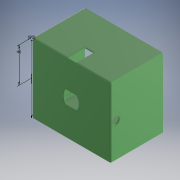
# Autodesk Inventor part: corps
Saved by Autodesk Inventor 2017 (Build 210142000, 142)
## iProperties
Part Number: corps
Material: Plastique ABS
Document SubType Name: Modeling
Designer: starl
Density: 1.06 g/cm^3
Appearance: Lisse - Blanc
Author: starl
Autodesk Inventor part; units mm, degrees
ref_plane "YZ Plane" through (0, 0, 0) normal (1, 0, 0) x (0, 1, 0)
ref_plane "XZ Plane" through (0, 0, 0) normal (0, 1, 0) x (-1, 0, 0)
ref_plane "XY Plane" through (0, 0, 0) normal (0, 0, 1) x (1, 0, 0)
sketch "Esquisse1" plane through (0, 0, 0) normal (1, 0, 0) x (0, 1, 0)
  line L0 (0, 0) -> (60, 0)
  line L1 (60, 0) -> (60, -80)
  line L2 (60, -80) -> (0, -80)
  line L3 (0, -80) -> (0, 0)
  line L4 (0, -45) -> (0, -35)
  line L5 (0, -35) -> (0, -45)
  point P0 (12.5, -45)
  point P1 (0, -40)
  point P2 (0, -40)
  dimension "d0" = 80
  dimension "d1" = 60
  dimension "d4" = 40
  constraints: 12 end point, 3 equal length, 3 midpoint, 1 horizontal, 1 perpendicular, 1 point on line
  measures "d0" distance of L0.end L1.end
  measures "d1" distance of L1.end L2.end
  measures "d4" distance of point (0, -40) L2.end
extrude "Extrusion1" add sketch "Esquisse1" along normal blind 90
sketch "Esquisse2" plane through (0, 0, 0) normal (-1, 0, 0) x (0, 0, 1)
  line L0 (0, 0) -> (-80, 0) projected
  line L1 (-45, 0) -> (-35, 0)
  line L2 (0, 0) -> (-80, 0) projected
  point P0 (-40, 0)
  point P1 (-40, 0)
  point P2 (-40, 1)
  point P3 (-41.0501, 0)
  point P4 (-35, 9.6008)
  point P5 (-45, 11)
  dimension "d9" = 40
  dimension "d14" = 80
  constraints: 3 midpoint, 2 end point, 2 point on line, 2 vertical alignment, 1 coincident, 1 horizontal
  measures "d9" distance of L0.start point (-40, 0)
  measures "d14" distance of L0.start L0.end
shell "Coque1" thickness 1 removed faces 1 at (30, 60, -53.3333)
sketch "Esquisse3" plane through (0, 0, 0) normal (-1, 0, 0) x (0, 0, 1)
  point P0 (0, 0)
sketch "Esquisse4" plane through (0, 0, 0) normal (-1, 0, 0) x (0, 0, 1)
  point P0 (0, 0)
sketch "Esquisse5" plane through (0, 0, -80) normal (0, 0, -1) x (-1, 0, 0)
  line L0 (-50.2889, 1) -> (-40.2889, 1)
  line L1 (-40.2889, 1) -> (-40.2889, 21)
  line L2 (-40.2889, 21) -> (-50.2889, 21)
  line L3 (-50.2889, 21) -> (-50.2889, 1)
  line L4 (0, 0) -> (-90, 0) projected
  line L5 (0, 0) -> (-90, 0) projected
  line L6 (-1, 1) -> (-89, 1) projected
  point P0 (-45, 0)
  point P1 (-40.2889, 0)
  point P2 (-49.4557, 1)
  point P3 (-46.3284, -7.001)
  point P4 (-44.591, 0)
  point P5 (-46.3284, -7.537)
  point P6 (-50.2889, 11)
  point P7 (-50.2889, 11)
  point P8 (-49.5179, 0)
  point P9 (-49.2163, 0)
  dimension "d15" = 10
  dimension "d16" = 20
  dimension "d17" = 1
  dimension "d18" = 88
  dimension "d19" = 90
  constraints: 8 end point, 6 point on line, 2 midpoint, 2 parallel, 1 coincident, 1 horizontal, 1 perpendicular
  measures "d15" distance of L1.end L2.end
  measures "d16" distance of L0.end L1.end
  measures "d17" distance between parallel lines of L4 L0
  measures "d18" distance of L6.start L6.end
  measures "d19" angle of L6 L1
sketch "Esquisse8" plane through (0, 0, 0) normal (0, 0, 1) x (1, 0, 0)
  point P0 (0, 0)
extrude "Extrusion2" cut sketch "Esquisse5" against normal blind 90
sketch "Esquisse9" plane through (0, 0, 0) normal (-1, 0, 0) x (0, 0, 1)
  line L0 (-50.5224, 1) -> (-50.5224, 2)
  line L1 (-66.5224, 2) -> (-66.5224, 1)
  line L2 (-70.063, 25) -> (-54.063, 25)
  line L3 (-54.063, 25) -> (-54.063, 11)
  line L4 (-54.063, 11) -> (-70.063, 11)
  line L5 (-70.063, 11) -> (-70.063, 25)
  line L6 (0, 0) -> (-80, 0) projected
  dimension "d23" = 1
  dimension "d24" = 11
  dimension "d25" = 14
  dimension "d26" = 16
  constraints: 12 end point, 3 parallel, 1 horizontal, 1 perpendicular
  measures "d23" distance of L0.start L0.end
  measures "d24" distance between parallel lines of L6 L4
  measures "d25" distance of L2.end L3.end
  measures "d26" distance of L2.start L2.end
extrude "Extrusion3" cut sketch "Esquisse9" against normal blind 50
sketch "Esquisse10" plane through (90, 0, 0) normal (1, 0, 0) x (0, 0, -1)
  circle A0 centre (39.7201, 6) radius 4.1979
  line L0 (0, 0) -> (80, 0) projected
  dimension "d29" = 6
  constraints: 1 centre point
  measures "d29" distance from line of L0 A0.centre
extrude "Extrusion4" cut sketch "Esquisse10" against normal blind 50
sketch "Esquisse11" plane through (0, 0, -80) normal (0, -1, 0) x (1, 0, 0)
  line L0 (39.1611, 33.4845) -> (51.1611, 33.4845)
  line L1 (51.1611, 33.4845) -> (51.1611, 48.4845)
  line L2 (51.1611, 48.4845) -> (39.1611, 48.4845)
  line L3 (39.1611, 48.4845) -> (39.1611, 33.4845)
  arc A0 (39.1611, 48.4845) -> (39.1611, 33.4845) centre (48.6459, 40.9845) ccw
  arc A1 (51.1611, 33.4845) -> (51.1611, 48.4845) centre (41.7255, 40.9845) ccw
  point P0 (0, 80)
  point P1 (36.5541, 40.9845)
  point P2 (53.7787, 40.9845)
  point P3 (45.1019, 41.2499)
  point P4 (27.4865, 33.4896)
  point P5 (27.0422, 33.4896)
  dimension "d32" = 15
  dimension "d33" = 12
  dimension "d34" = 6.9205
  dimension "d35" = 12.0918
  constraints: 8 end point, 6 point on circle, 2 centre point, 2 parallel, 1 horizontal, 1 perpendicular
  measures "d32" distance of L2.end L0.start
  measures "d33" distance of L1.end L2.end
  measures "d34" distance of A1.centre A0.centre
  measures "d35" radius of A0
extrude "Extrusion5" cut sketch "Esquisse11" against normal blind 10
fillet "Congé1" radius 2 2 edges at (1, 30.5, -79) (45, 0, -80)
fillet "Congé2" radius 2 2 edges at (90, 30, 0) (45, 0, 0)
fillet "Congé3" radius 2 5 edges at (90, 0.5858, -79.4142) (90, 31, -80) (89.4142, 0.5858, -0.5858) (90, 0, -40) (89, 30.5, -1)
fillet "Congé4" radius 2 5 edges at (0, 0.5858, -79.4142) (0, 31, -80) (0, 0.5858, -0.5858) (0, 31, 0) (0, 0, -40)
